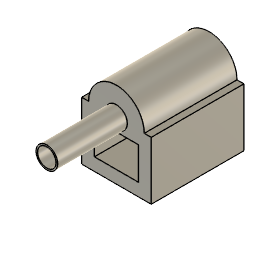
servo part (Autodesk Fusion 360 design; units mm, degrees)
part number: 2025-11-07-09-40-13-047
Autodesk Fusion 360 part; units mm, degrees
sketch "Sketch1" plane through (0, 0, 0) normal (0, 1, 0) x (1, 0, 0)
  line L0 (-7.5, 6.25) -> (7.5, 6.25)
  line L1 (7.5, 6.25) -> (7.5, -6.25)
  line L2 (-7.5, -6.25) -> (-7.5, 6.25)
  line L3 (-7.5, 6.25) -> (7.5, -6.25) construction
  line L4 (7.5, 6.25) -> (-7.5, -6.25) construction
  line L5 (7.5, -6.25) -> (6, -6.25)
  line L6 (-6, -6.25) -> (-7.5, -6.25)
  arc A0 (-6, -6.25) -> (6, -6.25) centre (0, -6.25) ccw
  arc A1 (0.3096, -0.258) -> (-0.3096, -0.258) centre (0, -6.25) ccw
  dimension "d1" = 15
  dimension "d2" = 12.5
  dimension "d3" = 12
  constraint horizontal L0
  constraint perpendicular L0 L1
  constraint parallel L0 L5
  constraint parallel L1 L2
  constraint coincident L3 origin
  constraint coincident L4 origin
  constraint coincident L4 A1.end
  constraint collinear L5 L6
  constraint coincident A0.centre L5
  constraint coincident L3 A1.start
  constraint concentric A0 A1
  measures "d1" distance of L1.end L2.start
  measures "d2" distance of L0.end L1.end
  measures "d3" diameter of A0
extrude "Extrude1" add sketch "Sketch1" along normal blind 20
sketch "Sketch2" plane through (0, 0, 0) normal (0, -1, 0) x (1, 0, 0)
  line L0 (-6, 6.25) -> (-7.5, 6.25)
  line L1 (-7.5, 6.25) -> (-7.5, -6.25)
  line L2 (-7.5, -6.25) -> (7.5, -6.25)
  line L3 (7.5, -6.25) -> (7.5, 6.25)
  line L4 (7.5, 6.25) -> (6, 6.25)
  arc A0 (6, 6.25) -> (-6, 6.25) centre (0, 6.25) ccw
  line L5 (4.75, -3.5) -> (-4.75, -3.5)
  line L6 (-4.75, -3.5) -> (-4.75, 3.5)
  line L7 (-4.75, 3.5) -> (4.75, 3.5)
  line L8 (4.75, 3.5) -> (4.75, -3.5)
  line L9 (4.75, -3.5) -> (-4.75, 3.5) construction
  line L10 (-4.75, -3.5) -> (4.75, 3.5) construction
  dimension "d6" = 9.5
  dimension "d7" = 7
  constraint horizontal L5
  constraint perpendicular L5 L6
  constraint parallel L5 L7
  constraint parallel L6 L8
  constraint coincident L9 origin
  constraint coincident L10 origin
  measures "d6" distance of L6.end L7.end
  measures "d7" distance of L5.end L6.end
extrude "Extrude2" cut sketch "Sketch2" against normal blind 39 contours L5 L6 L7 L8
sketch "Sketch3" plane through (0, 0, 0) normal (0, -1, 0) x (1, 0, 0)
  line L0 (-4.75, -3.5) -> (-4.75, 3.5)
  line L1 (-4.75, 3.5) -> (4.75, 3.5)
  line L2 (4.75, 3.5) -> (4.75, -3.5)
  line L3 (4.75, -3.5) -> (-4.75, -3.5)
  line L4 (-6, 6.25) -> (-7.5, 6.25)
  line L5 (-7.5, 6.25) -> (-7.5, -6.25)
  line L6 (-7.5, -6.25) -> (7.5, -6.25)
  line L7 (7.5, -6.25) -> (7.5, 6.25)
  line L8 (7.5, 6.25) -> (6, 6.25)
  arc A0 (6, 6.25) -> (-6, 6.25) centre (0, 6.25) ccw
  circle A1 centre (0, 6.25) radius 2
  dimension "d10" = 4
  constraint concentric A0 A1
  measures "d10" diameter of A1
extrude "Extrude3" cut sketch "Sketch3" against normal blind 30 contours A1
sketch "Sketch4" plane through (0, 0, 0) normal (0, -1, 0) x (1, 0, 0)
  circle A0 centre (0, 6.25) radius 2
  line L0 (-4.75, -3.5) -> (-4.75, 3.5)
  line L1 (-4.75, 3.5) -> (4.75, 3.5)
  line L2 (4.75, 3.5) -> (4.75, -3.5)
  line L3 (4.75, -3.5) -> (-4.75, -3.5)
  line L4 (-6, 6.25) -> (-7.5, 6.25)
  line L5 (-7.5, 6.25) -> (-7.5, -6.25)
  line L6 (-7.5, -6.25) -> (7.5, -6.25)
  line L7 (7.5, -6.25) -> (7.5, 6.25)
  line L8 (7.5, 6.25) -> (6, 6.25)
  arc A1 (6, 6.25) -> (-6, 6.25) centre (0, 6.25) ccw
  circle A2 centre (0, 6.25) radius 2.35
  dimension "d13" = 0.35
extrude "Extrude4" add sketch "Sketch4" along normal blind 15 contours A2
